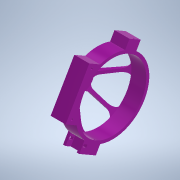
# Autodesk Inventor part: Prindere
Saved by Autodesk Inventor 2020.3 (Build 243373000, 373)
## iProperties
Created: 2021-03-16
Part Number: Prindere
Material: ABS Plastic
Document SubType Name: Modeling
Designer: alexo
Density: 1.06 g/cm^3
Appearance: Smooth - Purple
Mass: 115.773 g
Surface Area: 455.551 cm^2
Volume: 109.22 cm^3
Author: alexo
Autodesk Inventor part; units mm, degrees
sketch "Prindere" plane through (0, 0, 0) normal (0, 0, 1) x (1, 0, 0)
  arc A0 (63.8454, 123.0776) -> (56.3454, 123.0776) centre (60.0954, 123.0776) ccw construction
  line L0 (63.8454, 123.0776) -> (63.8454, 118.8276) construction
  arc A1 (63.8454, 118.8276) -> (71.8454, 110.8276) centre (71.8454, 118.8276) ccw construction
  line L1 (71.8454, 110.8276) -> (76.0954, 110.8276) construction
  arc A2 (76.0954, 103.3276) -> (76.0954, 110.8276) centre (76.0954, 107.0776) ccw construction
  line L2 (76.0954, 103.3276) -> (71.8454, 103.3276) construction
  arc A3 (71.8454, 103.3276) -> (63.8454, 95.3276) centre (71.8454, 95.3276) ccw construction
  line L3 (63.8454, 95.3276) -> (63.8454, 91.0776) construction
  arc A4 (56.3454, 91.0776) -> (63.8454, 91.0776) centre (60.0954, 91.0776) ccw construction
  line L4 (56.3454, 91.0776) -> (56.3454, 95.3276) construction
  arc A5 (56.3454, 95.3276) -> (48.3454, 103.3276) centre (48.3454, 95.3276) ccw construction
  line L5 (48.3454, 103.3276) -> (44.0954, 103.3276) construction
  arc A6 (44.0954, 110.8276) -> (44.0954, 103.3276) centre (44.0954, 107.0776) ccw construction
  line L6 (44.0954, 110.8276) -> (48.3454, 110.8276) construction
  arc A7 (48.3454, 110.8276) -> (56.3454, 118.8276) centre (48.3454, 118.8276) ccw construction
  line L7 (56.3454, 118.8276) -> (56.3454, 123.0776) construction
  circle A8 centre (60.0954, 123.0776) radius 1.5 construction
  circle A9 centre (60.0954, 107.0776) radius 5 construction
  circle A10 centre (44.0954, 107.0776) radius 1.5 construction
  circle A11 centre (60.0954, 91.0776) radius 1.5 construction
  circle A12 centre (76.0954, 107.0776) radius 1.5 construction
  point P0 (60.0954, 107.0776)
  dimension "d0" = 45
sketch "Sketch1" plane through (0, 0, 0) normal (1, 0, 0) x (0, 1, 0)
  circle A0 centre (0, 0) radius 22.5
  line L0 (0, 22.5) -> (0, -22.5) construction
  circle A1 centre (0, 16) radius 2
  circle A2 centre (-16, 0) radius 2
  circle A3 centre (0, -16) radius 2
  circle A4 centre (16, 0) radius 2
  circle A5 centre (0, 0) radius 6
  arc A6 (3.75, 16) -> (-3.75, 16) centre (0, 16) ccw construction
  line L1 (3.75, 16) -> (3.75, 11.75) construction
  arc A7 (3.75, 11.75) -> (11.75, 3.75) centre (11.75, 11.75) ccw construction
  line L2 (11.75, 3.75) -> (16, 3.75) construction
  arc A8 (16, -3.75) -> (16, 3.75) centre (16, 0) ccw construction
  line L3 (16, -3.75) -> (11.75, -3.75) construction
  arc A9 (11.75, -3.75) -> (3.75, -11.75) centre (11.75, -11.75) ccw construction
  line L4 (3.75, -11.75) -> (3.75, -16) construction
  arc A10 (-3.75, -16) -> (3.75, -16) centre (0, -16) ccw construction
  line L5 (-3.75, -16) -> (-3.75, -11.75) construction
  arc A11 (-3.75, -11.75) -> (-11.75, -3.75) centre (-11.75, -11.75) ccw construction
  line L6 (-11.75, -3.75) -> (-16, -3.75) construction
  arc A12 (-16, 3.75) -> (-16, -3.75) centre (-16, 0) ccw construction
  line L7 (-16, 3.75) -> (-11.75, 3.75) construction
  arc A13 (-11.75, 3.75) -> (-3.75, 11.75) centre (-11.75, 11.75) ccw construction
  line L8 (-3.75, 11.75) -> (-3.75, 16) construction
  circle A14 centre (0, 16) radius 1.5 construction
  circle A15 centre (0, 0) radius 5 construction
  circle A16 centre (-16, 0) radius 1.5 construction
  circle A17 centre (0, -16) radius 1.5 construction
  circle A18 centre (16, 0) radius 1.5 construction
  dimension "d0" = 45
  dimension "d1" = 4
  dimension "d2" = 4
  dimension "d3" = 4
  dimension "d4" = 4
  dimension "d5" = 12
  constraints: 6 centre point, 2 end point, 2 point on circle, 2 vertical, 1 coincident, 1 midpoint, 6 other
  measures "d0" diameter of A0
  measures "d1" diameter of A1
  measures "d2" diameter of A2
  measures "d3" diameter of A3
  measures "d4" diameter of A4
  measures "d5" diameter of A5
extrude "Extrusion1" add sketch "Sketch1" along normal blind 10
ref_plane "Work Plane1" through (0, 0, -16) normal (0, -1, 0) x (1, 0, 0)
sketch "Sketch3" plane through (0, 0, -16) normal (0, -1, 0) x (1, 0, 0)
  line L0 (0, -6.5) -> (10, -6.5) projected
  line L1 (10, -6.5) -> (40, -51.5)
  line L2 (10, -6.5) -> (10, 38.5) projected
  line L3 (0, 16) -> (40, 16) construction
  line L4 (40, 16) -> (40, -51.5) construction
  line L5 (10, -6.5) -> (0, 8.5)
  line L6 (0, -6.5) -> (0, 38.5) projected
  line L7 (0, 8.5) -> (0, -6.5)
  line L8 (0, -6.5) -> (40, -57.5)
  line L9 (40, -57.5) -> (40, -51.5)
  dimension "d8" = 30
  dimension "d9" = 67.5
  dimension "d17" = 6
  constraints: 14 end point, 1 collinear, 1 horizontal, 1 parallel, 1 perpendicular, 1 point on line, 1 vertical
  measures "d8" distance from line of L2 L1.end
  measures "d9" distance from line of L3 L1.end
  measures "d17" distance of L8.end L1.end
ref_plane "Work Plane2" through (0, 0, -22.5) normal (0, 0, -1) x (-1, 0, 0)
extrude "Extrusion2" add sketch "Sketch3" along normal mid plane 6
pattern_circular "Circular Pattern1" count 6 over 360 about axis through (0, 0, 0) along (1, 0, 0) of "Extrusion2"
sketch "Sketch5" plane through (40, 56.9567, -36.3481) normal (1, 0, 0) x (0, -0.5, -0.8660254)
  circle A0 centre (-3, -67.5) radius 6 projected
  circle A1 centre (-3, -67.5) radius 67.5
  line L0 (53.9567, -31.1519) -> (56.9567, -36.3481) projected
  circle A2 centre (-3, -67.5) radius 73.5
  line L1 (-65.1529, -28.1519) -> (-68.1529, -33.3481) projected
  point P0 (-66.6529, -30.75)
  constraints: 2 coincident, 1 centre point, 1 midpoint, 1 tangent, 3 other
extrude "Extrusion3" add sketch "Sketch5" along normal blind 30 contours A2
sketch "Sketch6" plane through (10, 0, 0) normal (1, 0, 0) x (0, 0, -1)
  circle A0 centre (0, -16) radius 2 projected
  circle A1 centre (0, 0) radius 6 projected
  circle A2 centre (16, 0) radius 2 projected
  circle A3 centre (0, 16) radius 2 projected
  circle A4 centre (-16, 0) radius 2 projected
extrude "Extrusion4" cut sketch "Sketch6" against normal through all
fillet "Fillet1" radius 10 12 edges at (40, -3, 70.4694) (40, 3, 70.4694) (40, 59.5283, 37.8328) (40, 62.5283, 32.6366) (40, -59.5283, 37.8328) (40, -62.5283, 32.6366) (40, -62.5283, -32.6366) (40, -59.5283, -37.8328) (40, -3, -70.4694) (40, 3, -70.4694) (40, 59.5283, -37.8328) (40, 62.5283, -32.6366)
fillet "Fillet2" radius 10 12 edges at (4.933, 3, -22.2991) (4.933, -3, -22.2991) (4.933, -17.8116, -13.7476) (4.933, -20.8116, -8.5515) (4.933, -17.8116, 13.7476) (4.933, -20.8116, 8.5515) (4.933, -3, 22.2991) (4.933, 3, 22.2991) (4.933, 17.8116, 13.7476) (4.933, 20.8116, 8.5515) (4.933, 20.8116, -8.5515) (4.933, 17.8116, -13.7476)
sketch "Sketch8" plane through (70, 0, 0) normal (1, 0, 0) x (0, 0, -1)
  circle A0 centre (0, 0) radius 73.5 projected
  arc A1 (-72.3412, -13) -> (-47.4289, -56.1493) centre (0, 0) ccw projected
  line L0 (-47.4289, -56.1493) -> (-56.2583, -71.4423)
  line L1 (-56.2583, -71.4423) -> (-33.7417, -84.4423)
  line L2 (-33.7417, -84.4423) -> (-24.9123, -69.1493)
  line L3 (-28.8481, -43.9663) -> (-17.4914, -24.2961) projected
  dimension "d24" = 90
  constraints: 6 end point, 2 parallel, 1 perpendicular
  measures "d24" distance from line of A0.centre L1
extrude "Extrusion6" add sketch "Sketch8" against normal up to surface (30 mm away) contours L2 L1 L0 A0
ref_plane "Work Plane3" through (40, -77.9423, 45) normal (-0.9659258, 0.1294095, 0.2241439) x (0, 0.8660254, -0.5)
sketch "Sketch9" plane through (40, -77.9423, 45) normal (-0.9659258, 0.1294095, 0.2241439) x (0, 0.8660254, -0.5)
  line L0 (-61.9356, 0) -> (232.4593, 0) projected
  line L1 (16.5, -2.8978) -> (16.5, 2.8978) projected
  circle A0 centre (15, 0) radius 3.25
  point P0 (90, 10.3528)
  dimension "d28" = 6.5
  dimension "d29" = 1.5
  constraints: 1 centre point, 1 point on line
  measures "d28" diameter of A0
  measures "d29" distance from line of L1 A0.centre
extrude "Extrusion7" cut sketch "Sketch9" against normal mid plane 30
pattern_circular "Circular Pattern2" count 2 over 360 about axis through (0, 0, 0) along (1, 0, 0) of "Extrusion6", "Extrusion7"
sketch "Sketch10" plane through (70, 56.9567, -36.3481) normal (1, 0, 0) x (0, -0.5, -0.8660254)
  arc A0 (-16, 4.8412) -> (-16, -139.8412) centre (-3, -67.5) ccw projected
  line L0 (-59.1493, -114.9289) -> (-84.5, -114.9289)
  line L1 (-84.5, -114.9289) -> (-84.5, -20.0711)
  line L2 (-84.5, -20.0711) -> (-59.1493, -20.0711)
  point P0 (-76.5, -67.5)
  dimension "d36" = 8
  constraints: 6 end point, 1 horizontal, 1 parallel, 1 perpendicular, 1 point on circle
  measures "d36" distance from line of L1 point (-76.5, -67.5)
extrude "Extrusion8" add sketch "Sketch10" against normal up to surface (30 mm away)
sketch "Sketch11" plane through (40, 56.9567, -36.3481) normal (-1, 0, 0) x (0, 0.5, 0.8660254)
  line L0 (59.1493, -114.9289) -> (84.5, -114.9289) projected
  line L1 (74.5, -114.9289) -> (74.5, -20.0711) construction
  line L2 (59.1493, -20.0711) -> (84.5, -20.0711) projected
  circle A0 centre (74.5, -106.9289) radius 2
  circle A1 centre (74.5, -28.0711) radius 2
  circle A2 centre (74.5, -106.9289) radius 4 construction
  line L3 (84.5, -114.9289) -> (84.5, -20.0711) projected
  line L4 (84.5, -20.0711) -> (59.1493, -20.0711) projected
  point P0 (3, -67.5)
  dimension "d39" = 4
  dimension "d40" = 4
  dimension "d41" = 8
  dimension "d42" = 8
  dimension "d43" = 8
  dimension "d47" = 10
  constraints: 4 point on line, 3 centre point, 2 end point, 1 coincident
  measures "d39" diameter of A0
  measures "d40" diameter of A1
  measures "d41" diameter of A2
  measures "d42" distance of L1.start A0.centre
  measures "d43" distance from line of L2 A1.centre
  measures "d47" distance between parallel lines of L3 L1
extrude "Extrusion9" cut sketch "Sketch11" against normal through all
sketch "Sketch12" plane through (40, -84.4423, 33.7417) normal (0, -0.8660254, 0.5) x (1, 0, 0)
  line L0 (30, 26) -> (30, 0) construction
  line L1 (30, 13) -> (0, 13) construction
  line L2 (0, 0) -> (0, 26) construction
  circle A0 centre (27, 13) radius 1.25
  point P0 (-40, 13)
  dimension "d48" = 2.5
  dimension "d49" = 3
  constraints: 2 end point, 2 midpoint, 1 centre point, 1 point on line
  measures "d48" diameter of A0
  measures "d49" distance of L1.start A0.centre
extrude "Extrusion10" cut sketch "Sketch12" against normal through all
sketch "Sketch13" plane through (40, -71.4423, 56.2583) normal (0, 0.5, 0.8660254) x (1, 0, 0)
  line L0 (25.1, 15.1) -> (25.1, 0)
  line L1 (0, 0) -> (0, 17.6588) construction
  line L2 (30, 0) -> (0, 0) projected
  line L3 (30, 17.6588) -> (30, 0) projected
  line L4 (0, 17.6588) -> (30, 17.6588) projected
  line L5 (25.1, 15.1) -> (25.1, 17.6588)
  line L6 (0, 17.6588) -> (30, 17.6588) projected
  point P0 (-40, 90)
  point P1 (25.1, 17.6588)
  point P2 (25.1, 0)
  constraints: 4 end point, 1 perpendicular, 1 point on line
ref_plane "Work Plane6" through (37.8, -66.5846, 67.772) normal (0, 0.5, 0.8660254) x (1, 0, 0)
extrude "Extrusion11" add sketch "Sketch13" along normal up to surface (12.4 mm away)
sketch "Sketch14" plane through (40, -84.4423, 33.7417) normal (-1, 0, 0) x (0, 0.5, 0.8660254)
  line L0 (38.4, 0) -> (0, 0) projected
  line L1 (26, 0) -> (26, 17.6588) projected
  line L2 (22, 0) -> (26, 0)
  line L3 (26, 0) -> (26, 17.6588)
  line L4 (26, 17.6588) -> (22, 17.6588)
  line L5 (22, 17.6588) -> (22, 0)
  point P0 (13, 90)
  dimension "d54" = 4
  constraints: 8 end point, 2 parallel, 1 horizontal, 1 perpendicular, 1 point on line
  measures "d54" distance between parallel lines of L1 L5
ref_plane "Work Plane7" through (37.6, -73.4207, 56.4315) normal (-1, 0, 0) x (0, 0.5, 0.8660254)
extrude "Extrusion12" add sketch "Sketch14" along normal up to surface (2.4 mm away)
sketch "Sketch15" plane through (37.6, -71.4423, 56.2583) normal (0, 0.5, 0.8660254) x (1, 0, 0)
  line L0 (0, 17.6588) -> (0, 0) projected
  line L1 (27.5, 0) -> (0, 0) projected
  line L2 (0, 17.6588) -> (4.9, 17.6588)
  line L3 (4.9, 17.6588) -> (4.9, 0)
  line L4 (4.9, 0) -> (0, 0)
  line L5 (0, 0) -> (0, 17.6588)
  point P0 (-37.6, 90)
  point P1 (4.9, 15.1)
  constraints: 8 end point, 2 parallel, 2 point on line, 1 horizontal, 1 perpendicular, 1 other
ref_plane "Work Plane8" through (37.8, -66.5846, 67.772) normal (0, 0.5, 0.8660254) x (1, 0, 0)
extrude "Extrusion13" add sketch "Sketch15" along normal up to surface (12.4 mm away)
sketch "Sketch16" plane through (40, -84.4423, 33.7417) normal (0, -0.8660254, 0.5) x (1, 0, 0)
  arc A0 (-1.4, 31.55) -> (-1.4, 32.85) centre (-0.6401, 32.2) ccw construction
  arc A1 (29, 32.85) -> (29, 31.55) centre (28.2401, 32.2) ccw construction
  circle A2 centre (28.2401, 32.2) radius 1.25
  circle A3 centre (-0.6401, 32.2) radius 1.25
  point P0 (-40, 13)
  dimension "d59" = 2.5
  dimension "d60" = 2.5
  constraints: 2 centre point, 2 coincident
  measures "d59" diameter of A2
  measures "d60" diameter of A3
extrude "Extrusion14" cut sketch "Sketch16" against normal blind 10
sketch "Sketch17" plane through (65.1, -49.9493, 58.1676) normal (0, 0.8660254, -0.5) x (1, 0, 0)
  line L0 (0, 0) -> (4.9, 0) projected
  line L1 (4.9, 12.4) -> (4.9, 0) projected
  line L2 (0, 12.4) -> (4.9, 12.4) projected
  line L3 (0, 12.4) -> (0, 0) projected
  arc A0 (-25.1, 12.4) -> (-25.9348, 16.4) centre (-35.1, 12.4) ccw projected
  line L4 (-25.9348, 16.4) -> (-27.5, 16.4) projected
  line L5 (-27.5, 16.4) -> (-27.5, 0) projected
  line L6 (-27.5, 0) -> (-22.6, 0) projected
  line L7 (-22.6, 12.4) -> (-22.6, 0) projected
  line L8 (-25.1, 12.4) -> (-22.6, 12.4) projected
  point P0 (-65.1, 25.4)
extrude "Extrusion15" add sketch "Sketch17" along normal blind 4.25
sketch "Sketch18" plane through (37.6, -73.4423, 52.7942) normal (-1, 0, 0) x (0, 0.5, 0.8660254)
  line L0 (16.3, 15.2) -> (4.1, 15.2) projected
  line L1 (14.2, 15.2) -> (6.2, 15.2)
  line L2 (6.2, 15.2) -> (6.2, 10.2)
  line L3 (6.2, 10.2) -> (14.2, 10.2)
  line L4 (14.2, 10.2) -> (14.2, 15.2)
  point P0 (-9, 90)
  point P1 (10.2, 15.2)
  point P2 (6.2, 15.2)
  dimension "d65" = 5
  dimension "d66" = 8
  constraints: 8 end point, 2 midpoint, 2 parallel, 1 horizontal, 1 perpendicular, 1 point on line
  measures "d65" distance of L3.end L1.start
  measures "d66" distance between parallel lines of L2 L4
extrude "Extrusion16" cut sketch "Sketch18" against normal through all
equation "\"d8\" = Gr"
equation "\"d9\" = 0.5 * Di"
equation "\"d17\" = th"
equation "\"d10\" = th"
equation "\"Gr\" = 30"
equation "\"Di\" = 135"
equation "\"th\" = 6"
equation "\"UnghiM\" = 15deg"
equation "\"d27\" = UnghiM"
body "Solid1"
